Autodesk Fusion 360 part; units mm, degrees
note: some values were not read from the file. Chosen so that the rebuilt part matches the saved one: which bodies a step acts on; which pieces of a blend or face edit are solid. Set by a fixed rule: which sketch regions a step uses.
(part 2 of 4)
  spline S17 degree 5 poles (12.1174, 16.1235) (12.1106, 16.126) (12.0971, 16.1308) (12.0768, 16.138) (12.0498, 16.1475) (12.0159, 16.1592) (11.9821, 16.1707) (11.9483, 16.1819) (11.9145, 16.193) (11.8807, 16.2039) (11.8468, 16.2146) (11.813, 16.225) (11.7792, 16.2353) (11.7454, 16.2454) (11.7116, 16.2552) (11.6778, 16.2649) (11.644, 16.2743) (11.6102, 16.2836) (11.5765, 16.2926) (11.5427, 16.3014) (11.509, 16.31) (11.4752, 16.3184) (11.4415, 16.3266) (11.4078, 16.3346) (11.3741, 16.3423) (11.3405, 16.3499) (11.3068, 16.3572) (11.2732, 16.3643) (11.2396, 16.3712) (11.206, 16.3778) (11.1724, 16.3842) (11.1389, 16.3904) (11.1054, 16.3964) (11.0719, 16.4021) (11.0384, 16.4076) (11.005, 16.4129) (10.9716, 16.418) (10.9382, 16.4228) (10.9049, 16.4273) (10.8716, 16.4316) (10.8383, 16.4357) (10.8051, 16.4395) (10.7719, 16.4431) (10.7388, 16.4464) (10.7057, 16.4495) (10.6726, 16.4523) (10.6396, 16.4548) (10.6066, 16.4571) (10.5737, 16.4591) (10.5409, 16.4608) (10.508, 16.4623) (10.4753, 16.4635) (10.4426, 16.4643) (10.41, 16.4649) (10.3774, 16.4651) (10.345, 16.465) (10.3125, 16.4647) (10.2802, 16.4641) (10.2479, 16.4632) (10.2156, 16.462) (10.1835, 16.4604) (10.1515, 16.4583) (10.1196, 16.4557) (10.0879, 16.4527) (10.0562, 16.4492) (10.0246, 16.4454) (9.9932, 16.4414) (9.9617, 16.4371) (9.9304, 16.4325) (9.8993, 16.4274) (9.8685, 16.4212) (9.8441, 16.4151) (9.8261, 16.4098) (9.8141, 16.4059) (9.8082, 16.4039) knots -1 -1 -1 -1 -1 -1 -0.98571429 -0.97142857 -0.95714286 -0.94285714 -0.92857143 -0.91428571 -0.9 -0.88571429 -0.87142857 -0.85714286 -0.84285714 -0.82857143 -0.81428571 -0.8 -0.78571429 -0.77142857 -0.75714286 -0.74285714 -0.72857143 -0.71428571 -0.7 -0.68571429 -0.67142857 -0.65714286 -0.64285714 -0.62857143 -0.61428571 -0.6 -0.58571429 -0.57142857 -0.55714286 -0.54285714 -0.52857143 -0.51428571 -0.5 -0.48571429 -0.47142857 -0.45714286 -0.44285714 -0.42857143 -0.41428571 -0.4 -0.38571429 -0.37142857 -0.35714286 -0.34285714 -0.32857143 -0.31428571 -0.3 -0.28571429 -0.27142857 -0.25714286 -0.24285714 -0.22857143 -0.21428571 -0.2 -0.18571429 -0.17142857 -0.15714286 -0.14285714 -0.12857143 -0.11428571 -0.1 -0.08571429 -0.07142857 -0.05714286 -0.04285714 -0.02857143 -0.01428571 0 0 0 0 0 0
  line L17 (9.8082, 16.4039) -> (9.5546, 16.3173)
  arc A36 (8.5618, 16.7569) -> (9.5546, 16.3173) centre (9.2961, 17.0744) ccw
  arc A37 (8.5618, 16.7569) -> (8.4802, 16.94) centre (0, 13.0546) ccw
  arc A38 (8.8179, 17.9719) -> (8.4802, 16.94) centre (9.2075, 17.2732) ccw
  line L18 (8.8179, 17.9719) -> (9.0519, 18.1024)
  spline S18 degree 5 poles (9.0519, 18.1024) (9.0574, 18.1055) (9.0683, 18.1117) (9.0843, 18.1216) (9.1051, 18.1357) (9.1304, 18.1544) (9.1551, 18.1741) (9.1794, 18.1943) (9.2036, 18.2148) (9.2276, 18.2355) (9.2516, 18.2564) (9.2753, 18.2776) (9.2989, 18.2992) (9.3221, 18.3211) (9.3451, 18.3435) (9.3678, 18.3663) (9.3902, 18.3895) (9.4125, 18.4129) (9.4346, 18.4365) (9.4566, 18.4604) (9.4783, 18.4845) (9.5, 18.5088) (9.5214, 18.5334) (9.5426, 18.5583) (9.5637, 18.5834) (9.5845, 18.6088) (9.6052, 18.6344) (9.6258, 18.6602) (9.6461, 18.6862) (9.6663, 18.7124) (9.6864, 18.7389) (9.7062, 18.7655) (9.726, 18.7924) (9.7455, 18.8194) (9.7649, 18.8467) (9.7841, 18.8741) (9.8032, 18.9017) (9.8221, 18.9296) (9.8409, 18.9576) (9.8595, 18.9858) (9.8779, 19.0141) (9.8962, 19.0427) (9.9144, 19.0714) (9.9324, 19.1003) (9.9502, 19.1294) (9.9679, 19.1586) (9.9854, 19.188) (10.0028, 19.2176) (10.02, 19.2474) (10.0371, 19.2773) (10.054, 19.3073) (10.0708, 19.3375) (10.0875, 19.3679) (10.1039, 19.3985) (10.1203, 19.4291) (10.1364, 19.46) (10.1525, 19.491) (10.1684, 19.5221) (10.1841, 19.5534) (10.1997, 19.5848) (10.2151, 19.6164) (10.2304, 19.6481) (10.2455, 19.68) (10.2605, 19.712) (10.2754, 19.7441) (10.2901, 19.7764) (10.3046, 19.8088) (10.319, 19.8413) (10.3333, 19.874) (10.3474, 19.9068) (10.3614, 19.9398) (10.3724, 19.9662) (10.3806, 19.9861) (10.3861, 19.9994) (10.3888, 20.0061) knots 0 0 0 0 0 0 0.01428571 0.02857143 0.04285714 0.05714286 0.07142857 0.08571429 0.1 0.11428571 0.12857143 0.14285714 0.15714286 0.17142857 0.18571429 0.2 0.21428571 0.22857143 0.24285714 0.25714286 0.27142857 0.28571429 0.3 0.31428571 0.32857143 0.34285714 0.35714286 0.37142857 0.38571429 0.4 0.41428571 0.42857143 0.44285714 0.45714286 0.47142857 0.48571429 0.5 0.51428571 0.52857143 0.54285714 0.55714286 0.57142857 0.58571429 0.6 0.61428571 0.62857143 0.64285714 0.65714286 0.67142857 0.68571429 0.7 0.71428571 0.72857143 0.74285714 0.75714286 0.77142857 0.78571429 0.8 0.81428571 0.82857143 0.84285714 0.85714286 0.87142857 0.88571429 0.9 0.91428571 0.92857143 0.94285714 0.95714286 0.97142857 0.98571429 1 1 1 1 1 1
  arc A39 (10.3888, 20.0061) -> (9.8216, 20.7868) centre (0, 13.0546) ccw
  spline S19 degree 5 poles (9.8216, 20.7868) (9.8144, 20.7863) (9.8001, 20.7852) (9.7786, 20.7835) (9.75, 20.7812) (9.7144, 20.7781) (9.6788, 20.7748) (9.6433, 20.7714) (9.6079, 20.7677) (9.5726, 20.7639) (9.5374, 20.7599) (9.5022, 20.7557) (9.4671, 20.7514) (9.4322, 20.7468) (9.3973, 20.7421) (9.3625, 20.7371) (9.3278, 20.732) (9.2931, 20.7267) (9.2586, 20.7212) (9.2242, 20.7156) (9.1899, 20.7097) (9.1556, 20.7037) (9.1215, 20.6974) (9.0875, 20.691) (9.0536, 20.6844) (9.0197, 20.6776) (8.986, 20.6706) (8.9524, 20.6634) (8.9189, 20.656) (8.8855, 20.6484) (8.8522, 20.6406) (8.8191, 20.6326) (8.786, 20.6245) (8.7531, 20.6161) (8.7203, 20.6075) (8.6876, 20.5987) (8.6551, 20.5897) (8.6226, 20.5805) (8.5903, 20.5712) (8.5581, 20.5616) (8.5261, 20.5517) (8.4942, 20.5417) (8.4624, 20.5315) (8.4308, 20.521) (8.3993, 20.5104) (8.368, 20.4995) (8.3368, 20.4884) (8.3057, 20.477) (8.2748, 20.4655) (8.2441, 20.4537) (8.2135, 20.4417) (8.1831, 20.4294) (8.1529, 20.4169) (8.1229, 20.4041) (8.0931, 20.3911) (8.0634, 20.3779) (8.034, 20.3644) (8.0046, 20.3506) (7.9755, 20.3367) (7.9465, 20.3225) (7.9179, 20.3079) (7.8895, 20.293) (7.8614, 20.2777) (7.8336, 20.262) (7.8061, 20.2459) (7.7788, 20.2296) (7.7517, 20.2132) (7.7247, 20.1965) (7.698, 20.1796) (7.6717, 20.1622) (7.646, 20.144) (7.6262, 20.1285) (7.6119, 20.1164) (7.6025, 20.1079) (7.5979, 20.1037) knots -1 -1 -1 -1 -1 -1 -0.98571429 -0.97142857 -0.95714286 -0.94285714 -0.92857143 -0.91428571 -0.9 -0.88571429 -0.87142857 -0.85714286 -0.84285714 -0.82857143 -0.81428571 -0.8 -0.78571429 -0.77142857 -0.75714286 -0.74285714 -0.72857143 -0.71428571 -0.7 -0.68571429 -0.67142857 -0.65714286 -0.64285714 -0.62857143 -0.61428571 -0.6 -0.58571429 -0.57142857 -0.55714286 -0.54285714 -0.52857143 -0.51428571 -0.5 -0.48571429 -0.47142857 -0.45714286 -0.44285714 -0.42857143 -0.41428571 -0.4 -0.38571429 -0.37142857 -0.35714286 -0.34285714 -0.32857143 -0.31428571 -0.3 -0.28571429 -0.27142857 -0.25714286 -0.24285714 -0.22857143 -0.21428571 -0.2 -0.18571429 -0.17142857 -0.15714286 -0.14285714 -0.12857143 -0.11428571 -0.1 -0.08571429 -0.07142857 -0.05714286 -0.04285714 -0.02857143 -0.01428571 0 0 0 0 0 0
  line L19 (7.5979, 20.1037) -> (7.4015, 19.9214)
  arc A40 (6.3157, 19.9192) -> (7.4015, 19.9214) centre (6.8574, 20.5079) ccw
  arc A41 (6.3157, 19.9192) -> (6.1668, 20.0533) centre (0, 13.0546) ccw
  arc A42 (6.0555, 21.1333) -> (6.1668, 20.0533) centre (6.6957, 20.6535) ccw
  line L20 (6.0555, 21.1333) -> (6.2162, 21.3477)
  spline S20 degree 5 poles (6.2162, 21.3477) (6.22, 21.3528) (6.2274, 21.3629) (6.238, 21.3785) (6.2513, 21.3998) (6.2667, 21.4272) (6.2813, 21.4552) (6.2953, 21.4835) (6.3091, 21.5121) (6.3226, 21.5408) (6.336, 21.5697) (6.3491, 21.5987) (6.3618, 21.6279) (6.3741, 21.6575) (6.3859, 21.6873) (6.3974, 21.7173) (6.4085, 21.7476) (6.4194, 21.778) (6.4299, 21.8086) (6.4403, 21.8394) (6.4504, 21.8702) (6.4602, 21.9013) (6.4698, 21.9325) (6.4791, 21.9638) (6.4881, 21.9953) (6.4968, 22.027) (6.5053, 22.0588) (6.5136, 22.0907) (6.5216, 22.1228) (6.5294, 22.1549) (6.5369, 22.1872) (6.5443, 22.2197) (6.5514, 22.2522) (6.5582, 22.2849) (6.5649, 22.3177) (6.5713, 22.3505) (6.5774, 22.3836) (6.5834, 22.4167) (6.5891, 22.4499) (6.5947, 22.4832) (6.6, 22.5166) (6.6051, 22.5502) (6.61, 22.5838) (6.6147, 22.6175) (6.6191, 22.6513) (6.6234, 22.6852) (6.6274, 22.7192) (6.6313, 22.7533) (6.6349, 22.7875) (6.6384, 22.8218) (6.6416, 22.8561) (6.6447, 22.8905) (6.6475, 22.925) (6.6501, 22.9596) (6.6526, 22.9943) (6.6548, 23.0291) (6.6568, 23.0639) (6.6587, 23.0988) (6.6603, 23.1338) (6.6618, 23.1688) (6.6631, 23.204) (6.6641, 23.2392) (6.665, 23.2744) (6.6657, 23.3097) (6.6662, 23.3451) (6.6665, 23.3806) (6.6666, 23.4161) (6.6665, 23.4517) (6.6662, 23.4874) (6.6658, 23.5231) (6.6651, 23.5589) (6.6645, 23.5875) (6.6639, 23.609) (6.6634, 23.6234) (6.6632, 23.6306) knots 0 0 0 0 0 0 0.01428571 0.02857143 0.04285714 0.05714286 0.07142857 0.08571429 0.1 0.11428571 0.12857143 0.14285714 0.15714286 0.17142857 0.18571429 0.2 0.21428571 0.22857143 0.24285714 0.25714286 0.27142857 0.28571429 0.3 0.31428571 0.32857143 0.34285714 0.35714286 0.37142857 0.38571429 0.4 0.41428571 0.42857143 0.44285714 0.45714286 0.47142857 0.48571429 0.5 0.51428571 0.52857143 0.54285714 0.55714286 0.57142857 0.58571429 0.6 0.61428571 0.62857143 0.64285714 0.65714286 0.67142857 0.68571429 0.7 0.71428571 0.72857143 0.74285714 0.75714286 0.77142857 0.78571429 0.8 0.81428571 0.82857143 0.84285714 0.85714286 0.87142857 0.88571429 0.9 0.91428571 0.92857143 0.94285714 0.95714286 0.97142857 0.98571429 1 1 1 1 1 1
  arc A43 (6.6632, 23.6306) -> (5.8275, 24.1131) centre (0, 13.0546) ccw
  spline S21 degree 5 poles (5.8275, 24.1131) (5.8211, 24.1097) (5.8085, 24.1029) (5.7895, 24.0927) (5.7644, 24.0789) (5.7331, 24.0616) (5.7019, 24.0441) (5.6709, 24.0265) (5.6401, 24.0088) (5.6093, 23.9909) (5.5788, 23.9729) (5.5484, 23.9548) (5.5181, 23.9366) (5.488, 23.9182) (5.4581, 23.8997) (5.4283, 23.881) (5.3987, 23.8622) (5.3692, 23.8433) (5.3399, 23.8242) (5.3107, 23.8051) (5.2818, 23.7858) (5.2529, 23.7663) (5.2243, 23.7467) (5.1958, 23.727) (5.1675, 23.7072) (5.1394, 23.6872) (5.1115, 23.6671) (5.0837, 23.6468) (5.0561, 23.6265) (5.0287, 23.6059) (5.0014, 23.5853) (4.9744, 23.5645) (4.9475, 23.5436) (4.9208, 23.5226) (4.8944, 23.5014) (4.8681, 23.4801) (4.842, 23.4586) (4.8161, 23.437) (4.7904, 23.4153) (4.7649, 23.3935) (4.7396, 23.3715) (4.7145, 23.3493) (4.6897, 23.327) (4.665, 23.3046) (4.6406, 23.2821) (4.6164, 23.2594) (4.5924, 23.2365) (4.5687, 23.2136) (4.5452, 23.1905) (4.5219, 23.1672) (4.4988, 23.1438) (4.4761, 23.1202) (4.4536, 23.0965) (4.4313, 23.0726) (4.4094, 23.0486) (4.3877, 23.0244) (4.3662, 23.0001) (4.345, 22.9756) (4.3241, 22.951) (4.3034, 22.9263) (4.2831, 22.9013) (4.2633, 22.8761) (4.2438, 22.8507) (4.2249, 22.8251) (4.2063, 22.7992) (4.188, 22.7733) (4.1699, 22.7472) (4.152, 22.721) (4.1345, 22.6946) (4.1175, 22.668) (4.1015, 22.641) (4.0897, 22.6188) (4.0815, 22.6019) (4.0764, 22.5904) (4.0739, 22.5846) knots -1 -1 -1 -1 -1 -1 -0.98571429 -0.97142857 -0.95714286 -0.94285714 -0.92857143 -0.91428571 -0.9 -0.88571429 -0.87142857 -0.85714286 -0.84285714 -0.82857143 -0.81428571 -0.8 -0.78571429 -0.77142857 -0.75714286 -0.74285714 -0.72857143 -0.71428571 -0.7 -0.68571429 -0.67142857 -0.65714286 -0.64285714 -0.62857143 -0.61428571 -0.6 -0.58571429 -0.57142857 -0.55714286 -0.54285714 -0.52857143 -0.51428571 -0.5 -0.48571429 -0.47142857 -0.45714286 -0.44285714 -0.42857143 -0.41428571 -0.4 -0.38571429 -0.37142857 -0.35714286 -0.34285714 -0.32857143 -0.31428571 -0.3 -0.28571429 -0.27142857 -0.25714286 -0.24285714 -0.22857143 -0.21428571 -0.2 -0.18571429 -0.17142857 -0.15714286 -0.14285714 -0.12857143 -0.11428571 -0.1 -0.08571429 -0.07142857 -0.05714286 -0.04285714 -0.02857143 -0.01428571 0 0 0 0 0 0
  line L21 (4.0739, 22.5846) -> (3.9686, 22.3382)
  arc A44 (2.9776, 21.8945) -> (3.9686, 22.3382) centre (3.233, 22.6527) ccw
  arc A45 (2.9776, 21.8945) -> (2.787, 21.9565) centre (0, 13.0546) ccw
  arc A46 (2.2461, 22.8979) -> (2.787, 21.9565) centre (3.026, 22.7199) ccw
  line L22 (2.2461, 22.8979) -> (2.3057, 23.1591)
  spline S22 degree 5 poles (2.3057, 23.1591) (2.3071, 23.1653) (2.3097, 23.1776) (2.3131, 23.1961) (2.3166, 23.2209) (2.3195, 23.2522) (2.3214, 23.2837) (2.3227, 23.3154) (2.3236, 23.347) (2.3244, 23.3788) (2.3248, 23.4106) (2.325, 23.4424) (2.3247, 23.4743) (2.3239, 23.5063) (2.3226, 23.5383) (2.3209, 23.5705) (2.3187, 23.6026) (2.3162, 23.6348) (2.3135, 23.6671) (2.3104, 23.6994) (2.3071, 23.7317) (2.3034, 23.764) (2.2995, 23.7964) (2.2952, 23.8288) (2.2906, 23.8613) (2.2858, 23.8938) (2.2806, 23.9263) (2.2751, 23.9588) (2.2694, 23.9913) (2.2634, 24.0239) (2.2572, 24.0565) (2.2507, 24.0891) (2.244, 24.1217) (2.2369, 24.1543) (2.2297, 24.187) (2.2221, 24.2196) (2.2144, 24.2523) (2.2063, 24.285) (2.1981, 24.3177) (2.1896, 24.3504) (2.1808, 24.3831) (2.1719, 24.4158) (2.1627, 24.4485) (2.1532, 24.4812) (2.1435, 24.5139) (2.1336, 24.5466) (2.1235, 24.5793) (2.1132, 24.612) (2.1026, 24.6447) (2.0918, 24.6774) (2.0808, 24.7101) (2.0696, 24.7428) (2.0581, 24.7755) (2.0465, 24.8082) (2.0346, 24.8408) (2.0225, 24.8735) (2.0102, 24.9061) (1.9977, 24.9388) (1.985, 24.9714) (1.972, 25.004) (1.9589, 25.0366) (1.9455, 25.0692) (1.932, 25.1018) (1.9183, 25.1343) (1.9043, 25.1669) (1.8902, 25.1994) (1.8758, 25.2319) (1.8613, 25.2644) (1.8465, 25.2968) (1.8316, 25.3292) (1.8164, 25.3617) (1.8042, 25.3876) (1.7949, 25.407) (1.7886, 25.42) (1.7855, 25.4264) knots 0 0 0 0 0 0 0.01428571 0.02857143 0.04285714 0.05714286 0.07142857 0.08571429 0.1 0.11428571 0.12857143 0.14285714 0.15714286 0.17142857 0.18571429 0.2 0.21428571 0.22857143 0.24285714 0.25714286 0.27142857 0.28571429 0.3 0.31428571 0.32857143 0.34285714 0.35714286 0.37142857 0.38571429 0.4 0.41428571 0.42857143 0.44285714 0.45714286 0.47142857 0.48571429 0.5 0.51428571 0.52857143 0.54285714 0.55714286 0.57142857 0.58571429 0.6 0.61428571 0.62857143 0.64285714 0.65714286 0.67142857 0.68571429 0.7 0.71428571 0.72857143 0.74285714 0.75714286 0.77142857 0.78571429 0.8 0.81428571 0.82857143 0.84285714 0.85714286 0.87142857 0.88571429 0.9 0.91428571 0.92857143 0.94285714 0.95714286 0.97142857 0.98571429 1 1 1 1 1 1
  arc A47 (1.7855, 25.4264) -> (0.8258, 25.5273) centre (0, 13.0546) ccw
  spline S23 degree 5 poles (0.8258, 25.5273) (0.8214, 25.5216) (0.8126, 25.5103) (0.7994, 25.4932) (0.782, 25.4704) (0.7605, 25.4418) (0.7391, 25.4132) (0.718, 25.3845) (0.697, 25.3558) (0.6762, 25.327) (0.6556, 25.2981) (0.6352, 25.2692) (0.615, 25.2402) (0.5949, 25.2111) (0.5751, 25.182) (0.5555, 25.1529) (0.5361, 25.1237) (0.5168, 25.0944) (0.4978, 25.0651) (0.479, 25.0357) (0.4604, 25.0063) (0.442, 24.9768) (0.4238, 24.9473) (0.4058, 24.9177) (0.388, 24.888) (0.3704, 24.8583) (0.3531, 24.8286) (0.3359, 24.7988) (0.319, 24.769) (0.3023, 24.7391) (0.2858, 24.7091) (0.2695, 24.6792) (0.2535, 24.6491) (0.2377, 24.619) (0.2221, 24.5889) (0.2068, 24.5588) (0.1917, 24.5286) (0.1768, 24.4983) (0.1622, 24.468) (0.1478, 24.4377) (0.1336, 24.4073) (0.1197, 24.3769) (0.1061, 24.3464) (0.0927, 24.3159) (0.0795, 24.2854) (0.0667, 24.2548) (0.054, 24.2242) (0.0417, 24.1935) (0.0296, 24.1629) (0.0178, 24.1321) (0.0062, 24.1014) (-0.005, 24.0706) (-0.0159, 24.0398) (-0.0265, 24.0089) (-0.0368, 23.978) (-0.0467, 23.9471) (-0.0564, 23.9162) (-0.0659, 23.8852) (-0.075, 23.8542) (-0.0838, 23.8232) (-0.0922, 23.7921) (-0.1001, 23.7611) (-0.1075, 23.7299) (-0.1144, 23.6988) (-0.1209, 23.6676) (-0.127, 23.6364) (-0.133, 23.6052) (-0.1386, 23.574) (-0.1439, 23.5429) (-0.1486, 23.5117) (-0.1523, 23.4804) (-0.154, 23.4554) (-0.1546, 23.4366) (-0.1546, 23.424) (-0.1545, 23.4177) knots -1 -1 -1 -1 -1 -1 -0.98571429 -0.97142857 -0.95714286 -0.94285714 -0.92857143 -0.91428571 -0.9 -0.88571429 -0.87142857 -0.85714286 -0.84285714 -0.82857143 -0.81428571 -0.8 -0.78571429 -0.77142857 -0.75714286 -0.74285714 -0.72857143 -0.71428571 -0.7 -0.68571429 -0.67142857 -0.65714286 -0.64285714 -0.62857143 -0.61428571 -0.6 -0.58571429 -0.57142857 -0.55714286 -0.54285714 -0.52857143 -0.51428571 -0.5 -0.48571429 -0.47142857 -0.45714286 -0.44285714 -0.42857143 -0.41428571 -0.4 -0.38571429 -0.37142857 -0.35714286 -0.34285714 -0.32857143 -0.31428571 -0.3 -0.28571429 -0.27142857 -0.25714286 -0.24285714 -0.22857143 -0.21428571 -0.2 -0.18571429 -0.17142857 -0.15714286 -0.14285714 -0.12857143 -0.11428571 -0.1 -0.08571429 -0.07142857 -0.05714286 -0.04285714 -0.02857143 -0.01428571 0 0 0 0 0 0
  line L23 (-0.1545, 23.4177) -> (-0.1505, 23.1498)
  arc A48 (-0.8753, 22.3414) -> (-0.1505, 23.1498) centre (-0.9504, 23.1379) ccw
  arc A49 (-0.8753, 22.3414) -> (-1.0746, 22.3204) centre (0, 13.0546) ccw
  arc A50 (-1.9517, 22.9605) -> (-1.0746, 22.3204) centre (-1.1668, 23.1151) ccw
  line L24 (-1.9517, 22.9605) -> (-2.0035, 23.2234)
  spline S24 degree 5 poles (-2.0035, 23.2234) (-2.0047, 23.2295) (-2.0073, 23.2418) (-2.0118, 23.2601) (-2.0187, 23.2842) (-2.0288, 23.314) (-2.0398, 23.3436) (-2.0515, 23.373) (-2.0636, 23.4023) (-2.0758, 23.4316) (-2.0883, 23.4608) (-2.1011, 23.49) (-2.1144, 23.519) (-2.1281, 23.5479) (-2.1423, 23.5767) (-2.157, 23.6053) (-2.172, 23.6338) (-2.1874, 23.6622) (-2.203, 23.6906) (-2.219, 23.7188) (-2.2352, 23.747) (-2.2516, 23.7751) (-2.2684, 23.803) (-2.2855, 23.8309) (-2.3029, 23.8587) (-2.3205, 23.8864) (-2.3385, 23.914) (-2.3567, 23.9415) (-2.3751, 23.9689) (-2.3939, 23.9962) (-2.4128, 24.0234) (-2.432, 24.0506) (-2.4514, 24.0776) (-2.4711, 24.1046) (-2.491, 24.1314) (-2.5112, 24.1582) (-2.5316, 24.1849) (-2.5522, 24.2115) (-2.5731, 24.238) (-2.5941, 24.2644) (-2.6154, 24.2907) (-2.6369, 24.3169) (-2.6586, 24.343) (-2.6805, 24.3691) (-2.7027, 24.395) (-2.725, 24.4209) (-2.7476, 24.4467) (-2.7703, 24.4723) (-2.7933, 24.4979) (-2.8165, 24.5234) (-2.8398, 24.5488) (-2.8634, 24.5741) (-2.8871, 24.5993) (-2.9111, 24.6244) (-2.9352, 24.6494) (-2.9595, 24.6743) (-2.9841, 24.6991) (-3.0088, 24.7239) (-3.0337, 24.7485) (-3.0587, 24.773) (-3.084, 24.7975) (-3.1094, 24.8218) (-3.135, 24.846) (-3.1608, 24.8702) (-3.1868, 24.8942) (-3.213, 24.9182) (-3.2393, 24.9421) (-3.2658, 24.9658) (-3.2925, 24.9895) (-3.3193, 25.013) (-3.3463, 25.0365) (-3.3681, 25.0552) (-3.3845, 25.0691) (-3.3954, 25.0784) (-3.4009, 25.0831) knots 0 0 0 0 0 0 0.01428571 0.02857143 0.04285714 0.05714286 0.07142857 0.08571429 0.1 0.11428571 0.12857143 0.14285714 0.15714286 0.17142857 0.18571429 0.2 0.21428571 0.22857143 0.24285714 0.25714286 0.27142857 0.28571429 0.3 0.31428571 0.32857143 0.34285714 0.35714286 0.37142857 0.38571429 0.4 0.41428571 0.42857143 0.44285714 0.45714286 0.47142857 0.48571429 0.5 0.51428571 0.52857143 0.54285714 0.55714286 0.57142857 0.58571429 0.6 0.61428571 0.62857143 0.64285714 0.65714286 0.67142857 0.68571429 0.7 0.71428571 0.72857143 0.74285714 0.75714286 0.77142857 0.78571429 0.8 0.81428571 0.82857143 0.84285714 0.85714286 0.87142857 0.88571429 0.9 0.91428571 0.92857143 0.94285714 0.95714286 0.97142857 0.98571429 1 1 1 1 1 1
  arc A51 (-3.4009, 25.0831) -> (-4.3187, 24.7848) centre (0, 13.0546) ccw
  spline S25 degree 5 poles (-4.3187, 24.7848) (-4.3205, 24.7779) (-4.3239, 24.7639) (-4.3289, 24.743) (-4.3355, 24.7151) (-4.3436, 24.6802) (-4.3515, 24.6454) (-4.3591, 24.6106) (-4.3666, 24.5758) (-4.3739, 24.541) (-4.381, 24.5062) (-4.3879, 24.4715) (-4.3945, 24.4368) (-4.401, 24.4021) (-4.4073, 24.3675) (-4.4133, 24.3329) (-4.4192, 24.2983) (-4.4249, 24.2637) (-4.4303, 24.2292) (-4.4356, 24.1947) (-4.4406, 24.1603) (-4.4454, 24.1258) (-4.45, 24.0914) (-4.4544, 24.0571) (-4.4586, 24.0228) (-4.4626, 23.9885) (-4.4664, 23.9543) (-4.4699, 23.9201) (-4.4732, 23.886) (-4.4763, 23.8519) (-4.4792, 23.8178) (-4.4819, 23.7838) (-4.4843, 23.7498) (-4.4865, 23.7159) (-4.4885, 23.6821) (-4.4903, 23.6483) (-4.4918, 23.6145) (-4.4931, 23.5808) (-4.4941, 23.5472) (-4.4949, 23.5136) (-4.4955, 23.4801) (-4.4958, 23.4467) (-4.4959, 23.4133) (-4.4957, 23.38) (-4.4953, 23.3468) (-4.4946, 23.3136) (-4.4937, 23.2805) (-4.4925, 23.2475) (-4.4911, 23.2145) (-4.4894, 23.1817) (-4.4874, 23.1489) (-4.4852, 23.1162) (-4.4826, 23.0836) (-4.4797, 23.0511) (-4.4765, 23.0187) (-4.4731, 22.9864) (-4.4694, 22.9542) (-4.4654, 22.9221) (-4.4611, 22.89) (-4.4565, 22.8581) (-4.4516, 22.8263) (-4.4461, 22.7947) (-4.4403, 22.7633) (-4.4339, 22.732) (-4.4271, 22.7009) (-4.4201, 22.6699) (-4.4128, 22.639) (-4.4053, 22.6082) (-4.3974, 22.5776) (-4.389, 22.5471) (-4.3796, 22.5171) (-4.3711, 22.4935) (-4.3639, 22.4761) (-4.3588, 22.4647) (-4.3562, 22.4589) knots -1 -1 -1 -1 -1 -1 -0.98571429 -0.97142857 -0.95714286 -0.94285714 -0.92857143 -0.91428571 -0.9 -0.88571429 -0.87142857 -0.85714286 -0.84285714 -0.82857143 -0.81428571 -0.8 -0.78571429 -0.77142857 -0.75714286 -0.74285714 -0.72857143 -0.71428571 -0.7 -0.68571429 -0.67142857 -0.65714286 -0.64285714 -0.62857143 -0.61428571 -0.6 -0.58571429 -0.57142857 -0.55714286 -0.54285714 -0.52857143 -0.51428571 -0.5 -0.48571429 -0.47142857 -0.45714286 -0.44285714 -0.42857143 -0.41428571 -0.4 -0.38571429 -0.37142857 -0.35714286 -0.34285714 -0.32857143 -0.31428571 -0.3 -0.28571429 -0.27142857 -0.25714286 -0.24285714 -0.22857143 -0.21428571 -0.2 -0.18571429 -0.17142857 -0.15714286 -0.14285714 -0.12857143 -0.11428571 -0.1 -0.08571429 -0.07142857 -0.05714286 -0.04285714 -0.02857143 -0.01428571 0 0 0 0 0 0
  line L25 (-4.3562, 22.4589) -> (-4.2435, 22.2158)
  arc A52 (-4.5769, 21.1825) -> (-4.2435, 22.2158) centre (-4.9694, 21.8796) ccw
  arc A53 (-4.5769, 21.1825) -> (-4.7505, 21.0823) centre (0, 13.0546) ccw
  arc A54 (-5.8121, 21.3102) -> (-4.7505, 21.0823) centre (-5.1579, 21.7708) ccw
  line L26 (-5.8121, 21.3102) -> (-5.9663, 21.5293)
  spline S26 degree 5 poles (-5.9663, 21.5293) (-5.9699, 21.5345) (-5.9773, 21.5446) (-5.9888, 21.5595) (-6.005, 21.5788) (-6.0263, 21.6019) (-6.0484, 21.6244) (-6.071, 21.6465) (-6.0939, 21.6684) (-6.1171, 21.6902) (-6.1404, 21.7118) (-6.1639, 21.7332) (-6.1878, 21.7543) (-6.2121, 21.7751) (-6.2368, 21.7956) (-6.2618, 21.8158) (-6.2872, 21.8358) (-6.3128, 21.8555) (-6.3386, 21.875) (-6.3646, 21.8943) (-6.3909, 21.9134) (-6.4174, 21.9324) (-6.4441, 21.9511) (-6.471, 21.9697) (-6.4982, 21.988) (-6.5256, 22.0061) (-6.5532, 22.024) (-6.581, 22.0417) (-6.609, 22.0592) (-6.6372, 22.0766) (-6.6656, 22.0937) (-6.6942, 22.1107) (-6.723, 22.1275) (-6.7519, 22.1442) (-6.781, 22.1606) (-6.8103, 22.1768) (-6.8398, 22.1929) (-6.8695, 22.2088) (-6.8993, 22.2246) (-6.9293, 22.2401) (-6.9594, 22.2555) (-6.9897, 22.2707) (-7.0202, 22.2858) (-7.0508, 22.3006) (-7.0816, 22.3153) (-7.1125, 22.3299) (-7.1436, 22.3442) (-7.1748, 22.3584) (-7.2062, 22.3724) (-7.2377, 22.3863) (-7.2694, 22.4) (-7.3012, 22.4135) (-7.3332, 22.4269) (-7.3652, 22.4401) (-7.3975, 22.4531) (-7.4298, 22.466) (-7.4623, 22.4787) (-7.495, 22.4912) (-7.5277, 22.5036) (-7.5606, 22.5158) (-7.5936, 22.5279) (-7.6267, 22.5398) (-7.66, 22.5515) (-7.6934, 22.5631) (-7.7269, 22.5745) (-7.7606, 22.5857) (-7.7943, 22.5968) (-7.8282, 22.6077) (-7.8622, 22.6185) (-7.8963, 22.6291) (-7.9305, 22.6395) (-7.958, 22.6477) (-7.9786, 22.6538) (-7.9924, 22.6579) (-7.9993, 22.6599) knots 0 0 0 0 0 0 0.01428571 0.02857143 0.04285714 0.05714286 0.07142857 0.08571429 0.1 0.11428571 0.12857143 0.14285714 0.15714286 0.17142857 0.18571429 0.2 0.21428571 0.22857143 0.24285714 0.25714286 0.27142857 0.28571429 0.3 0.31428571 0.32857143 0.34285714 0.35714286 0.37142857 0.38571429 0.4 0.41428571 0.42857143 0.44285714 0.45714286 0.47142857 0.48571429 0.5 0.51428571 0.52857143 0.54285714 0.55714286 0.57142857 0.58571429 0.6 0.61428571 0.62857143 0.64285714 0.65714286 0.67142857 0.68571429 0.7 0.71428571 0.72857143 0.74285714 0.75714286 0.77142857 0.78571429 0.8 0.81428571 0.82857143 0.84285714 0.85714286 0.87142857 0.88571429 0.9 0.91428571 0.92857143 0.94285714 0.95714286 0.97142857 0.98571429 1 1 1 1 1 1
  arc A55 (-7.9993, 22.6599) -> (-8.7165, 22.0141) centre (0, 13.0546) ccw
  spline S27 degree 5 poles (-8.7165, 22.0141) (-8.7152, 22.0071) (-8.7126, 21.9929) (-8.7087, 21.9717) (-8.7034, 21.9436) (-8.6966, 21.9084) (-8.6896, 21.8734) (-8.6825, 21.8385) (-8.6752, 21.8036) (-8.6677, 21.7689) (-8.66, 21.7343) (-8.6522, 21.6998) (-8.6442, 21.6654) (-8.636, 21.631) (-8.6276, 21.5968) (-8.6191, 21.5628) (-8.6104, 21.5288) (-8.6015, 21.4949) (-8.5924, 21.4611) (-8.5832, 21.4275) (-8.5738, 21.394) (-8.5642, 21.3606) (-8.5544, 21.3273) (-8.5445, 21.2941) (-8.5343, 21.261) (-8.524, 21.2281) (-8.5135, 21.1953) (-8.5029, 21.1626) (-8.492, 21.1301) (-8.481, 21.0977) (-8.4698, 21.0654) (-8.4584, 21.0333) (-8.4468, 21.0013) (-8.435, 20.9694) (-8.423, 20.9376) (-8.4109, 20.9061) (-8.3985, 20.8746) (-8.386, 20.8433) (-8.3733, 20.8122) (-8.3604, 20.7812) (-8.3473, 20.7503) (-8.334, 20.7196) (-8.3205, 20.6891) (-8.3068, 20.6588) (-8.2929, 20.6286) (-8.2788, 20.5985) (-8.2645, 20.5687) (-8.2499, 20.539) (-8.2352, 20.5095) (-8.2203, 20.4801) (-8.2052, 20.451) (-8.1898, 20.422) (-8.1742, 20.3933) (-8.1584, 20.3648) (-8.1423, 20.3365) (-8.126, 20.3084) (-8.1095, 20.2805) (-8.0928, 20.2527) (-8.0759, 20.2252) (-8.0587, 20.1979) (-8.0412, 20.1709) (-8.0234, 20.1442) (-8.0053, 20.1179) (-7.9867, 20.0919) (-7.9679, 20.0663) (-7.9488, 20.0408) (-7.9296, 20.0156) (-7.9102, 19.9905) (-7.8906, 19.9657) (-7.8705, 19.9413) (-7.8498, 19.9177) (-7.8323, 19.8996) (-7.8187, 19.8866) (-7.8094, 19.8782) (-7.8046, 19.8741) knots -1 -1 -1 -1 -1 -1 -0.98571429 -0.97142857 -0.95714286 -0.94285714 -0.92857143 -0.91428571 -0.9 -0.88571429 -0.87142857 -0.85714286 -0.84285714 -0.82857143 -0.81428571 -0.8 -0.78571429 -0.77142857 -0.75714286 -0.74285714 -0.72857143 -0.71428571 -0.7 -0.68571429 -0.67142857 -0.65714286 -0.64285714 -0.62857143 -0.61428571 -0.6 -0.58571429 -0.57142857 -0.55714286 -0.54285714 -0.52857143 -0.51428571 -0.5 -0.48571429 -0.47142857 -0.45714286 -0.44285714 -0.42857143 -0.41428571 -0.4 -0.38571429 -0.37142857 -0.35714286 -0.34285714 -0.32857143 -0.31428571 -0.3 -0.28571429 -0.27142857 -0.25714286 -0.24285714 -0.22857143 -0.21428571 -0.2 -0.18571429 -0.17142857 -0.15714286 -0.14285714 -0.12857143 -0.11428571 -0.1 -0.08571429 -0.07142857 -0.05714286 -0.04285714 -0.02857143 -0.01428571 0 0 0 0 0 0
  line L27 (-7.8046, 19.8741) -> (-7.6029, 19.6978)
  arc A56 (-7.4871, 18.6182) -> (-7.6029, 19.6978) centre (-8.1292, 19.0953) ccw
  arc A57 (-7.4871, 18.6182) -> (-7.6049, 18.456) centre (0, 13.0546) ccw
  arc A58 (-8.6674, 18.2325) -> (-7.6049, 18.456) centre (-8.2572, 18.9193) ccw
  line L28 (-8.6674, 18.2325) -> (-8.8975, 18.3699)
  spline S28 degree 5 poles (-8.8975, 18.3699) (-8.9029, 18.3732) (-8.9137, 18.3794) (-8.9303, 18.3884) (-8.9529, 18.3994) (-8.9818, 18.4118) (-9.0111, 18.4234) (-9.0408, 18.4344) (-9.0706, 18.4451) (-9.1006, 18.4555) (-9.1307, 18.4658) (-9.1609, 18.4758) (-9.1914, 18.4854) (-9.222, 18.4945) (-9.2529, 18.5032) (-9.284, 18.5115) (-9.3152, 18.5194) (-9.3466, 18.527) (-9.3782, 18.5343) (-9.4098, 18.5413) (-9.4416, 18.5482) (-9.4735, 18.5547) (-9.5055, 18.5609) (-9.5376, 18.5669) (-9.5699, 18.5726) (-9.6023, 18.578) (-9.6348, 18.5831) (-9.6674, 18.588) (-9.7002, 18.5926) (-9.733, 18.597) (-9.7659, 18.6011) (-9.7989, 18.605) (-9.832, 18.6087) (-9.8652, 18.6121) (-9.8985, 18.6152) (-9.9319, 18.6182) (-9.9654, 18.6209) (-9.9989, 18.6233) (-10.0326, 18.6256) (-10.0663, 18.6276) (-10.1001, 18.6294) (-10.134, 18.631) (-10.1679, 18.6323) (-10.2019, 18.6334) (-10.236, 18.6344) (-10.2702, 18.635) (-10.3044, 18.6355) (-10.3387, 18.6358) (-10.3731, 18.6358) (-10.4075, 18.6357) (-10.442, 18.6353) (-10.4766, 18.6347) (-10.5112, 18.6339) (-10.5459, 18.6329) (-10.5806, 18.6317) (-10.6154, 18.6303) (-10.6503, 18.6287) (-10.6852, 18.6269) (-10.7202, 18.6249) (-10.7552, 18.6227) (-10.7902, 18.6203) (-10.8253, 18.6176) (-10.8605, 18.6148) (-10.8957, 18.6118) (-10.931, 18.6086) (-10.9663, 18.6052) (-11.0016, 18.6016) (-11.037, 18.5978) (-11.0724, 18.5938) (-11.1079, 18.5896) (-11.1434, 18.5852) (-11.1718, 18.5816) (-11.1932, 18.5787) (-11.2074, 18.5768) (-11.2145, 18.5758) knots 0 0 0 0 0 0 0.01428571 0.02857143 0.04285714 0.05714286 0.07142857 0.08571429 0.1 0.11428571 0.12857143 0.14285714 0.15714286 0.17142857 0.18571429 0.2 0.21428571 0.22857143 0.24285714 0.25714286 0.27142857 0.28571429 0.3 0.31428571 0.32857143 0.34285714 0.35714286 0.37142857 0.38571429 0.4 0.41428571 0.42857143 0.44285714 0.45714286 0.47142857 0.48571429 0.5 0.51428571 0.52857143 0.54285714 0.55714286 0.57142857 0.58571429 0.6 0.61428571 0.62857143 0.64285714 0.65714286 0.67142857 0.68571429 0.7 0.71428571 0.72857143 0.74285714 0.75714286 0.77142857 0.78571429 0.8 0.81428571 0.82857143 0.84285714 0.85714286 0.87142857 0.88571429 0.9 0.91428571 0.92857143 0.94285714 0.95714286 0.97142857 0.98571429 1 1 1 1 1 1
  arc A59 (-11.2145, 18.5758) -> (-11.6071, 17.6942) centre (0, 13.0546) ccw
  spline S29 degree 5 poles (-11.6071, 17.6942) (-11.603, 17.6883) (-11.5949, 17.6764) (-11.5827, 17.6586) (-11.5664, 17.6351) (-11.5459, 17.6057) (-11.5253, 17.5766) (-11.5046, 17.5476) (-11.4837, 17.5187) (-11.4628, 17.4901) (-11.4417, 17.4616) (-11.4205, 17.4332) (-11.3991, 17.405) (-11.3777, 17.377) (-11.3562, 17.3492) (-11.3345, 17.3215) (-11.3127, 17.294) (-11.2908, 17.2667) (-11.2688, 17.2395) (-11.2467, 17.2125) (-11.2244, 17.1857) (-11.2021, 17.1591) (-11.1796, 17.1327) (-11.157, 17.1064) (-11.1344, 17.0803) (-11.1115, 17.0545) (-11.0886, 17.0288) (-11.0656, 17.0032) (-11.0424, 16.9779) (-11.0192, 16.9528) (-10.9958, 16.9279) (-10.9723, 16.9031) (-10.9487, 16.8786) (-10.925, 16.8543) (-10.9011, 16.8302) (-10.8772, 16.8063) (-10.8531, 16.7825) (-10.829, 16.759) (-10.8047, 16.7358) (-10.7803, 16.7127) (-10.7558, 16.6898) (-10.7311, 16.6672) (-10.7064, 16.6448) (-10.6815, 16.6227) (-10.6565, 16.6007) (-10.6314, 16.5791) (-10.6062, 16.5576) (-10.5809, 16.5364) (-10.5554, 16.5154) (-10.5299, 16.4947) (-10.5042, 16.4742) (-10.4784, 16.454) (-10.4524, 16.4341) (-10.4264, 16.4145) (-10.4002, 16.3952) (-10.3738, 16.3761) (-10.3474, 16.3573) (-10.3209, 16.3388) (-10.2942, 16.3205) (-10.2674, 16.3026) (-10.2405, 16.285) (-10.2134, 16.2679) (-10.1861, 16.2512) (-10.1586, 16.235) (-10.1309, 16.2192) (-10.1032, 16.2037) (-10.0753, 16.1885) (-10.0474, 16.1735) (-10.0194, 16.1588) (-9.9912, 16.1447) (-9.9626, 16.1316) (-9.9393, 16.1221) (-9.9216, 16.1158) (-9.9096, 16.1119) (-9.9036, 16.1101) knots -1 -1 -1 -1 -1 -1 -0.98571429 -0.97142857 -0.95714286 -0.94285714 -0.92857143 -0.91428571 -0.9 -0.88571429 -0.87142857 -0.85714286 -0.84285714 -0.82857143 -0.81428571 -0.8 -0.78571429 -0.77142857 -0.75714286 -0.74285714 -0.72857143 -0.71428571 -0.7 -0.68571429 -0.67142857 -0.65714286 -0.64285714 -0.62857143 -0.61428571 -0.6 -0.58571429 -0.57142857 -0.55714286 -0.54285714 -0.52857143 -0.51428571 -0.5 -0.48571429 -0.47142857 -0.45714286 -0.44285714 -0.42857143 -0.41428571 -0.4 -0.38571429 -0.37142857 -0.35714286 -0.34285714 -0.32857143 -0.31428571 -0.3 -0.28571429 -0.27142857 -0.25714286 -0.24285714 -0.22857143 -0.21428571 -0.2 -0.18571429 -0.17142857 -0.15714286 -0.14285714 -0.12857143 -0.11428571 -0.1 -0.08571429 -0.07142857 -0.05714286 -0.04285714 -0.02857143 -0.01428571 0 0 0 0 0 0
  line L29 (-9.9036, 16.1101) -> (-9.6476, 16.0311)
  arc A60 (-9.1027, 15.0919) -> (-9.6476, 16.0311) centre (-9.8834, 15.2666) ccw
extrude "Extrude8" cut sketch "Sketch7" along normal blind 25 contours A0 bodies 1 makes body 2 at (-1.8603, -53.3333, 13.789)
delete_face "DeleteFace1" 1 faces at (-1.8603, -53.3333, 13.789) on bodies 2
move_body "Move6" bodies 1 to x (1, 0, 0) y (0, 1, 0) z (0, 0, 1) at (0, -25, 0)
copy_body "CopyPasteBodies1" bodies 1 makes body 3
move_body "Move7" bodies 3 to x (-1, 0, 0) y (0, -1, 0) z (0, 0, 1) at (-4, 10, 0)
move_body "Move8" bodies 3 to x (1, 0, 0) y (0, 1, 0) z (0, 0, 1) at (4, -10, 0)
extrude "Extrude9" cut 1 faces at (-0.1483, 5, 12.35) along direction (0, 1, 0) blind 30 on bodies 1 bodies 1
move_body "Move9" bodies 2 to x (1, 0, 0) y (0, 1, 0) z (0, 0, 1) at (0, 30, 0)
extrude "Extrude10" add 1 faces at (0.1483, -5, 12.35) along direction (0, 1, 0) blind 30 on bodies 3 bodies 2 3
move_body "Move10" bodies 1 to x (1, 0, 0) y (0, 1, 0) z (0, 0, 1) at (0, 4, 0)
extrude "Extrude11" cut 1 faces at (-0.551, 49, 11.9624) along direction (0, -1, 0) blind 10 on bodies 1 bodies 1
move_body "Move11" bodies 1 to x (1, 0, 0) y (0, 1, 0) z (0, 0, 1) at (0, 1, 0)
extrude "Extrude12" add 1 faces at (-0.2877, 40, 12.9616) along direction (0, -1, 0) blind 4 on bodies 1 bodies 1
sketch "Sketch8" plane through (0, 35, 0) normal (0, 1, 0) x (-1, 0, 0)
  arc A0 (-9.1027, 15.0919) -> (-9.1444, 14.8959) centre (0, 13.0546) ccw
  arc A1 (-10.0241, 14.2595) -> (-9.1444, 14.8959) centre (-9.9287, 15.0538) ccw
  line L0 (-10.0241, 14.2595) -> (-10.2902, 14.2915)
  spline S0 degree 5 poles (-10.2902, 14.2915) (-10.2964, 14.2922) (-10.3089, 14.2935) (-10.3277, 14.295) (-10.3528, 14.2958) (-10.3842, 14.2955) (-10.4157, 14.2941) (-10.4473, 14.2921) (-10.4789, 14.2897) (-10.5106, 14.2871) (-10.5422, 14.2842) (-10.5739, 14.281) (-10.6056, 14.2774) (-10.6373, 14.2733) (-10.6691, 14.2687) (-10.7008, 14.2636) (-10.7326, 14.2581) (-10.7644, 14.2522) (-10.7962, 14.2461) (-10.828, 14.2397) (-10.8597, 14.233) (-10.8915, 14.226) (-10.9233, 14.2187) (-10.9551, 14.211) (-10.9869, 14.2031) (-11.0187, 14.1948) (-11.0505, 14.1863) (-11.0823, 14.1775) (-11.114, 14.1684) (-11.1458, 14.1591) (-11.1776, 14.1494) (-11.2093, 14.1396) (-11.241, 14.1295) (-11.2727, 14.1191) (-11.3045, 14.1084) (-11.3361, 14.0975) (-11.3678, 14.0864) (-11.3995, 14.075) (-11.4311, 14.0633) (-11.4627, 14.0515) (-11.4943, 14.0394) (-11.5259, 14.027) (-11.5575, 14.0144) (-11.589, 14.0016) (-11.6206, 13.9886) (-11.6521, 13.9753) (-11.6835, 13.9618) (-11.715, 13.9481) (-11.7464, 13.9342) (-11.7778, 13.92) (-11.8091, 13.9057) (-11.8405, 13.8911) (-11.8718, 13.8763) (-11.9031, 13.8613) (-11.9343, 13.846) (-11.9655, 13.8306) (-11.9967, 13.815) (-12.0279, 13.7991) (-12.059, 13.783) (-12.0901, 13.7668) (-12.1211, 13.7503) (-12.1521, 13.7336) (-12.1831, 13.7168) (-12.214, 13.6997) (-12.2449, 13.6824) (-12.2758, 13.6649) (-12.3066, 13.6473) (-12.3374, 13.6294) (-12.3682, 13.6113) (-12.3988, 13.5931) (-12.4295, 13.5746) (-12.454, 13.5597) (-12.4723, 13.5485) (-12.4846, 13.5409) (-12.4907, 13.5371) knots 0 0 0 0 0 0 0.01428571 0.02857143 0.04285714 0.05714286 0.07142857 0.08571429 0.1 0.11428571 0.12857143 0.14285714 0.15714286 0.17142857 0.18571429 0.2 0.21428571 0.22857143 0.24285714 0.25714286 0.27142857 0.28571429 0.3 0.31428571 0.32857143 0.34285714 0.35714286 0.37142857 0.38571429 0.4 0.41428571 0.42857143 0.44285714 0.45714286 0.47142857 0.48571429 0.5 0.51428571 0.52857143 0.54285714 0.55714286 0.57142857 0.58571429 0.6 0.61428571 0.62857143 0.64285714 0.65714286 0.67142857 0.68571429 0.7 0.71428571 0.72857143 0.74285714 0.75714286 0.77142857 0.78571429 0.8 0.81428571 0.82857143 0.84285714 0.85714286 0.87142857 0.88571429 0.9 0.91428571 0.92857143 0.94285714 0.95714286 0.97142857 0.98571429 1 1 1 1 1 1
  arc A2 (-12.4907, 13.5371) -> (-12.4907, 12.5721) centre (0, 13.0546) ccw
  spline S1 degree 5 poles (-12.4907, 12.5721) (-12.4846, 12.5683) (-12.4723, 12.5608) (-12.454, 12.5495) (-12.4295, 12.5346) (-12.3988, 12.5161) (-12.3682, 12.4979) (-12.3374, 12.4798) (-12.3066, 12.4619) (-12.2758, 12.4443) (-12.2449, 12.4268) (-12.214, 12.4095) (-12.1831, 12.3925) (-12.1521, 12.3756) (-12.1211, 12.3589) (-12.0901, 12.3424) (-12.059, 12.3262) (-12.0279, 12.3101) (-11.9967, 12.2943) (-11.9655, 12.2786) (-11.9343, 12.2632) (-11.9031, 12.2479) (-11.8718, 12.2329) (-11.8405, 12.2181) (-11.8091, 12.2035) (-11.7778, 12.1892) (-11.7464, 12.175) (-11.715, 12.1611) (-11.6835, 12.1474) (-11.6521, 12.1339) (-11.6206, 12.1206) (-11.589, 12.1076) (-11.5575, 12.0948) (-11.5259, 12.0822) (-11.4943, 12.0699) (-11.4627, 12.0578) (-11.4311, 12.0459) (-11.3995, 12.0342) (-11.3678, 12.0229) (-11.3361, 12.0117) (-11.3045, 12.0008) (-11.2727, 11.9902) (-11.241, 11.9798) (-11.2093, 11.9696) (-11.1776, 11.9598) (-11.1458, 11.9502) (-11.114, 11.9408) (-11.0823, 11.9317) (-11.0505, 11.9229) (-11.0187, 11.9144) (-10.9869, 11.9061) (-10.9551, 11.8982) (-10.9233, 11.8905) (-10.8915, 11.8832) (-10.8597, 11.8762) (-10.828, 11.8696) (-10.7962, 11.8631) (-10.7644, 11.857) (-10.7326, 11.8512) (-10.7008, 11.8457) (-10.6691, 11.8406) (-10.6373, 11.8359) (-10.6056, 11.8318) (-10.5739, 11.8282) (-10.5422, 11.825) (-10.5106, 11.8222) (-10.4789, 11.8195) (-10.4473, 11.8172) (-10.4157, 11.8151) (-10.3842, 11.8138) (-10.3528, 11.8134) (-10.3277, 11.8143) (-10.3089, 11.8157) (-10.2964, 11.817) (-10.2902, 11.8177) knots -1 -1 -1 -1 -1 -1 -0.98571429 -0.97142857 -0.95714286 -0.94285714 -0.92857143 -0.91428571 -0.9 -0.88571429 -0.87142857 -0.85714286 -0.84285714 -0.82857143 -0.81428571 -0.8 -0.78571429 -0.77142857 -0.75714286 -0.74285714 -0.72857143 -0.71428571 -0.7 -0.68571429 -0.67142857 -0.65714286 -0.64285714 -0.62857143 -0.61428571 -0.6 -0.58571429 -0.57142857 -0.55714286 -0.54285714 -0.52857143 -0.51428571 -0.5 -0.48571429 -0.47142857 -0.45714286 -0.44285714 -0.42857143 -0.41428571 -0.4 -0.38571429 -0.37142857 -0.35714286 -0.34285714 -0.32857143 -0.31428571 -0.3 -0.28571429 -0.27142857 -0.25714286 -0.24285714 -0.22857143 -0.21428571 -0.2 -0.18571429 -0.17142857 -0.15714286 -0.14285714 -0.12857143 -0.11428571 -0.1 -0.08571429 -0.07142857 -0.05714286 -0.04285714 -0.02857143 -0.01428571 0 0 0 0 0 0
  line L1 (-10.2902, 11.8177) -> (-10.0241, 11.8497)
  arc A3 (-9.1444, 11.2134) -> (-10.0241, 11.8497) centre (-9.9287, 11.0554) ccw
  arc A4 (-9.1444, 11.2134) -> (-9.1027, 11.0173) centre (0, 13.0546) ccw
  arc A5 (-9.6476, 10.0781) -> (-9.1027, 11.0173) centre (-9.8834, 10.8426) ccw
  line L2 (-9.6476, 10.0781) -> (-9.9036, 9.9991)
  spline S2 degree 5 poles (-9.9036, 9.9991) (-9.9096, 9.9973) (-9.9216, 9.9934) (-9.9393, 9.9871) (-9.9626, 9.9777) (-9.9912, 9.9645) (-10.0194, 9.9505) (-10.0474, 9.9358) (-10.0753, 9.9207) (-10.1032, 9.9055) (-10.1309, 9.89) (-10.1586, 9.8742) (-10.1861, 9.858) (-10.2134, 9.8413) (-10.2405, 9.8242) (-10.2674, 9.8066) (-10.2942, 9.7887) (-10.3209, 9.7704) (-10.3474, 9.7519) (-10.3738, 9.7331) (-10.4002, 9.714) (-10.4264, 9.6947) (-10.4524, 9.6751) (-10.4784, 9.6552) (-10.5042, 9.635) (-10.5299, 9.6146) (-10.5554, 9.5938) (-10.5809, 9.5728) (-10.6062, 9.5516) (-10.6314, 9.5302) (-10.6565, 9.5085) (-10.6815, 9.4865) (-10.7064, 9.4644) (-10.7311, 9.442) (-10.7558, 9.4194) (-10.7803, 9.3965) (-10.8047, 9.3735) (-10.829, 9.3502) (-10.8531, 9.3267) (-10.8772, 9.303) (-10.9011, 9.279) (-10.925, 9.2549) (-10.9487, 9.2306) (-10.9723, 9.2061) (-10.9958, 9.1813) (-11.0192, 9.1564) (-11.0424, 9.1313) (-11.0656, 9.106) (-11.0886, 9.0805) (-11.1115, 9.0548) (-11.1344, 9.0289) (-11.157, 9.0028) (-11.1796, 8.9766) (-11.2021, 8.9501) (-11.2244, 8.9235) (-11.2467, 8.8967) (-11.2688, 8.8697) (-11.2908, 8.8426) (-11.3127, 8.8152) (-11.3345, 8.7877) (-11.3562, 8.7601) (-11.3777, 8.7322) (-11.3991, 8.7042) (-11.4205, 8.676) (-11.4417, 8.6477) (-11.4628, 8.6192) (-11.4837, 8.5905) (-11.5046, 8.5616) (-11.5253, 8.5326) (-11.5459, 8.5035) (-11.5664, 8.4742) (-11.5827, 8.4506) (-11.5949, 8.4328) (-11.603, 8.4209) (-11.6071, 8.415) knots 0 0 0 0 0 0 0.01428571 0.02857143 0.04285714 0.05714286 0.07142857 0.08571429 0.1 0.11428571 0.12857143 0.14285714 0.15714286 0.17142857 0.18571429 0.2 0.21428571 0.22857143 0.24285714 0.25714286 0.27142857 0.28571429 0.3 0.31428571 0.32857143 0.34285714 0.35714286 0.37142857 0.38571429 0.4 0.41428571 0.42857143 0.44285714 0.45714286 0.47142857 0.48571429 0.5 0.51428571 0.52857143 0.54285714 0.55714286 0.57142857 0.58571429 0.6 0.61428571 0.62857143 0.64285714 0.65714286 0.67142857 0.68571429 0.7 0.71428571 0.72857143 0.74285714 0.75714286 0.77142857 0.78571429 0.8 0.81428571 0.82857143 0.84285714 0.85714286 0.87142857 0.88571429 0.9 0.91428571 0.92857143 0.94285714 0.95714286 0.97142857 0.98571429 1 1 1 1 1 1
  arc A6 (-11.6071, 8.415) -> (-11.2145, 7.5334) centre (0, 13.0546) ccw
  spline S3 degree 5 poles (-11.2145, 7.5334) (-11.2074, 7.5324) (-11.1932, 7.5305) (-11.1718, 7.5277) (-11.1434, 7.524) (-11.1079, 7.5196) (-11.0724, 7.5154) (-11.037, 7.5114) (-11.0016, 7.5076) (-10.9663, 7.504) (-10.931, 7.5006) (-10.8957, 7.4974) (-10.8605, 7.4944) (-10.8253, 7.4916) (-10.7902, 7.489) (-10.7552, 7.4865) (-10.7202, 7.4843) (-10.6852, 7.4823) (-10.6503, 7.4805) (-10.6154, 7.4789) (-10.5806, 7.4775) (-10.5459, 7.4763) (-10.5112, 7.4753) (-10.4766, 7.4745) (-10.442, 7.4739) (-10.4075, 7.4735) (-10.3731, 7.4734) (-10.3387, 7.4734) (-10.3044, 7.4737) (-10.2702, 7.4742) (-10.236, 7.4749) (-10.2019, 7.4758) (-10.1679, 7.4769) (-10.134, 7.4783) (-10.1001, 7.4798) (-10.0663, 7.4816) (-10.0326, 7.4836) (-9.9989, 7.4859) (-9.9654, 7.4883) (-9.9319, 7.491) (-9.8985, 7.494) (-9.8652, 7.4971) (-9.832, 7.5006) (-9.7989, 7.5042) (-9.7659, 7.5081) (-9.733, 7.5122) (-9.7002, 7.5166) (-9.6674, 7.5212) (-9.6348, 7.5261) (-9.6023, 7.5312) (-9.5699, 7.5366) (-9.5376, 7.5423) (-9.5055, 7.5483) (-9.4735, 7.5545) (-9.4416, 7.5611) (-9.4098, 7.5679) (-9.3782, 7.5749) (-9.3466, 7.5823) (-9.3152, 7.5899) (-9.284, 7.5977) (-9.2529, 7.606) (-9.222, 7.6147) (-9.1914, 7.6238) (-9.1609, 7.6334) (-9.1307, 7.6434) (-9.1006, 7.6537) (-9.0706, 7.6642) (-9.0408, 7.6748) (-9.0111, 7.6858) (-8.9818, 7.6974) (-8.9529, 7.7099) (-8.9303, 7.7208) (-8.9137, 7.7298) (-8.9029, 7.7361) (-8.8975, 7.7393) knots -1 -1 -1 -1 -1 -1 -0.98571429 -0.97142857 -0.95714286 -0.94285714 -0.92857143 -0.91428571 -0.9 -0.88571429 -0.87142857 -0.85714286 -0.84285714 -0.82857143 -0.81428571 -0.8 -0.78571429 -0.77142857 -0.75714286 -0.74285714 -0.72857143 -0.71428571 -0.7 -0.68571429 -0.67142857 -0.65714286 -0.64285714 -0.62857143 -0.61428571 -0.6 -0.58571429 -0.57142857 -0.55714286 -0.54285714 -0.52857143 -0.51428571 -0.5 -0.48571429 -0.47142857 -0.45714286 -0.44285714 -0.42857143 -0.41428571 -0.4 -0.38571429 -0.37142857 -0.35714286 -0.34285714 -0.32857143 -0.31428571 -0.3 -0.28571429 -0.27142857 -0.25714286 -0.24285714 -0.22857143 -0.21428571 -0.2 -0.18571429 -0.17142857 -0.15714286 -0.14285714 -0.12857143 -0.11428571 -0.1 -0.08571429 -0.07142857 -0.05714286 -0.04285714 -0.02857143 -0.01428571 0 0 0 0 0 0
  line L3 (-8.8975, 7.7393) -> (-8.6674, 7.8767)
  arc A7 (-7.6049, 7.6532) -> (-8.6674, 7.8767) centre (-8.2572, 7.1899) ccw
  arc A8 (-7.6049, 7.6532) -> (-7.4871, 7.491) centre (0, 13.0546) ccw
  arc A9 (-7.6029, 6.4114) -> (-7.4871, 7.491) centre (-8.1292, 7.0139) ccw
  line L4 (-7.6029, 6.4114) -> (-7.8046, 6.2351)
  spline S4 degree 5 poles (-7.8046, 6.2351) (-7.8094, 6.231) (-7.8187, 6.2226) (-7.8323, 6.2096) (-7.8498, 6.1915) (-7.8705, 6.1679) (-7.8906, 6.1436) (-7.9102, 6.1187) (-7.9296, 6.0937) (-7.9488, 6.0684) (-7.9679, 6.043) (-7.9867, 6.0173) (-8.0053, 5.9913) (-8.0234, 5.965) (-8.0412, 5.9383) (-8.0587, 5.9113) (-8.0759, 5.884) (-8.0928, 5.8565) (-8.1095, 5.8287) (-8.126, 5.8008) (-8.1423, 5.7727) (-8.1584, 5.7444) (-8.1742, 5.7159) (-8.1898, 5.6872) (-8.2052, 5.6582) (-8.2203, 5.6291) (-8.2352, 5.5997) (-8.2499, 5.5702) (-8.2645, 5.5405) (-8.2788, 5.5107) (-8.2929, 5.4807) (-8.3068, 5.4505) (-8.3205, 5.4201) (-8.334, 5.3896) (-8.3473, 5.3589) (-8.3604, 5.3281) (-8.3733, 5.2971) (-8.386, 5.2659) (-8.3985, 5.2346) (-8.4109, 5.2032) (-8.423, 5.1716) (-8.435, 5.1398) (-8.4468, 5.108) (-8.4584, 5.076) (-8.4698, 5.0438) (-8.481, 5.0115) (-8.492, 4.9791) (-8.5029, 4.9466) (-8.5135, 4.9139) (-8.524, 4.8811) (-8.5343, 4.8482) (-8.5445, 4.8151) (-8.5544, 4.782) (-8.5642, 4.7487) (-8.5738, 4.7153) (-8.5832, 4.6817) (-8.5924, 4.6481) (-8.6015, 4.6143) (-8.6104, 4.5805) (-8.6191, 4.5465) (-8.6276, 4.5124) (-8.636, 4.4782) (-8.6442, 4.4439) (-8.6522, 4.4094) (-8.66, 4.3749) (-8.6677, 4.3403) (-8.6752, 4.3056) (-8.6825, 4.2707) (-8.6896, 4.2358) (-8.6966, 4.2008) (-8.7034, 4.1657) (-8.7087, 4.1375) (-8.7126, 4.1163) (-8.7152, 4.1022) (-8.7165, 4.0951) knots 0 0 0 0 0 0 0.01428571 0.02857143 0.04285714 0.05714286 0.07142857 0.08571429 0.1 0.11428571 0.12857143 0.14285714 0.15714286 0.17142857 0.18571429 0.2 0.21428571 0.22857143 0.24285714 0.25714286 0.27142857 0.28571429 0.3 0.31428571 0.32857143 0.34285714 0.35714286 0.37142857 0.38571429 0.4 0.41428571 0.42857143 0.44285714 0.45714286 0.47142857 0.48571429 0.5 0.51428571 0.52857143 0.54285714 0.55714286 0.57142857 0.58571429 0.6 0.61428571 0.62857143 0.64285714 0.65714286 0.67142857 0.68571429 0.7 0.71428571 0.72857143 0.74285714 0.75714286 0.77142857 0.78571429 0.8 0.81428571 0.82857143 0.84285714 0.85714286 0.87142857 0.88571429 0.9 0.91428571 0.92857143 0.94285714 0.95714286 0.97142857 0.98571429 1 1 1 1 1 1
  arc A10 (-8.7165, 4.0951) -> (-7.9993, 3.4494) centre (0, 13.0546) ccw
  spline S5 degree 5 poles (-7.9993, 3.4494) (-7.9924, 3.4514) (-7.9786, 3.4554) (-7.958, 3.4615) (-7.9305, 3.4697) (-7.8963, 3.4802) (-7.8622, 3.4908) (-7.8282, 3.5015) (-7.7943, 3.5124) (-7.7606, 3.5235) (-7.7269, 3.5348) (-7.6934, 3.5462) (-7.66, 3.5577) (-7.6267, 3.5695) (-7.5936, 3.5813) (-7.5606, 3.5934) (-7.5277, 3.6056) (-7.495, 3.618) (-7.4623, 3.6305) (-7.4298, 3.6432) (-7.3975, 3.6561) (-7.3652, 3.6691) (-7.3332, 3.6823) (-7.3012, 3.6957) (-7.2694, 3.7092) (-7.2377, 3.7229) (-7.2062, 3.7368) (-7.1748, 3.7508) (-7.1436, 3.765) (-7.1125, 3.7794) (-7.0816, 3.7939) (-7.0508, 3.8086) (-7.0202, 3.8235) (-6.9897, 3.8385) (-6.9594, 3.8537) (-6.9293, 3.8691) (-6.8993, 3.8847) (-6.8695, 3.9004) (-6.8398, 3.9163) (-6.8103, 3.9324) (-6.781, 3.9486) (-6.7519, 3.9651) (-6.723, 3.9817) (-6.6942, 3.9985) (-6.6656, 4.0155) (-6.6372, 4.0326) (-6.609, 4.05) (-6.581, 4.0675) (-6.5532, 4.0852) (-6.5256, 4.1031) (-6.4982, 4.1212) (-6.471, 4.1396) (-6.4441, 4.1581) (-6.4174, 4.1768) (-6.3909, 4.1958) (-6.3646, 4.2149) (-6.3386, 4.2342) (-6.3128, 4.2538) (-6.2872, 4.2735) (-6.2618, 4.2934) (-6.2368, 4.3136) (-6.2121, 4.3341) (-6.1878, 4.3549) (-6.1639, 4.376) (-6.1404, 4.3974) (-6.1171, 4.4191) (-6.0939, 4.4408) (-6.071, 4.4627) (-6.0484, 4.4848) (-6.0263, 4.5073) (-6.005, 4.5305) (-5.9888, 4.5497) (-5.9773, 4.5646) (-5.9699, 4.5747) (-5.9663, 4.5799) knots -1 -1 -1 -1 -1 -1 -0.98571429 -0.97142857 -0.95714286 -0.94285714 -0.92857143 -0.91428571 -0.9 -0.88571429 -0.87142857 -0.85714286 -0.84285714 -0.82857143 -0.81428571 -0.8 -0.78571429 -0.77142857 -0.75714286 -0.74285714 -0.72857143 -0.71428571 -0.7 -0.68571429 -0.67142857 -0.65714286 -0.64285714 -0.62857143 -0.61428571 -0.6 -0.58571429 -0.57142857 -0.55714286 -0.54285714 -0.52857143 -0.51428571 -0.5 -0.48571429 -0.47142857 -0.45714286 -0.44285714 -0.42857143 -0.41428571 -0.4 -0.38571429 -0.37142857 -0.35714286 -0.34285714 -0.32857143 -0.31428571 -0.3 -0.28571429 -0.27142857 -0.25714286 -0.24285714 -0.22857143 -0.21428571 -0.2 -0.18571429 -0.17142857 -0.15714286 -0.14285714 -0.12857143 -0.11428571 -0.1 -0.08571429 -0.07142857 -0.05714286 -0.04285714 -0.02857143 -0.01428571 0 0 0 0 0 0
  line L5 (-5.9663, 4.5799) -> (-5.8121, 4.799)
  arc A11 (-4.7505, 5.0269) -> (-5.8121, 4.799) centre (-5.1579, 4.3385) ccw
  arc A12 (-4.7505, 5.0269) -> (-4.5769, 4.9267) centre (0, 13.0546) ccw
  arc A13 (-4.2435, 3.8934) -> (-4.5769, 4.9267) centre (-4.9694, 4.2297) ccw
  line L6 (-4.2435, 3.8934) -> (-4.3562, 3.6503)
  spline S6 degree 5 poles (-4.3562, 3.6503) (-4.3588, 3.6446) (-4.3639, 3.6331) (-4.3711, 3.6157) (-4.3796, 3.5921) (-4.389, 3.5621) (-4.3974, 3.5317) (-4.4053, 3.501) (-4.4128, 3.4702) (-4.4201, 3.4393) (-4.4271, 3.4083) (-4.4339, 3.3772) (-4.4403, 3.3459) (-4.4461, 3.3145) (-4.4516, 3.2829) (-4.4565, 3.2511) (-4.4611, 3.2192) (-4.4654, 3.1872) (-4.4694, 3.155) (-4.4731, 3.1228) (-4.4765, 3.0905) (-4.4797, 3.0581) (-4.4826, 3.0256) (-4.4852, 2.993) (-4.4874, 2.9603) (-4.4894, 2.9276) (-4.4911, 2.8947) (-4.4925, 2.8617) (-4.4937, 2.8287) (-4.4946, 2.7956) (-4.4953, 2.7624) (-4.4957, 2.7292) (-4.4959, 2.6959) (-4.4958, 2.6625) (-4.4955, 2.6291) (-4.4949, 2.5956) (-4.4941, 2.562) (-4.4931, 2.5284) (-4.4918, 2.4947) (-4.4903, 2.4609) (-4.4885, 2.4271) (-4.4865, 2.3933) (-4.4843, 2.3594) (-4.4819, 2.3254) (-4.4792, 2.2914) (-4.4763, 2.2574) (-4.4732, 2.2233) (-4.4699, 2.1891) (-4.4664, 2.1549) (-4.4626, 2.1207) (-4.4586, 2.0864) (-4.4544, 2.0521) (-4.45, 2.0178) (-4.4454, 1.9834) (-4.4406, 1.949) (-4.4356, 1.9145) (-4.4303, 1.88) (-4.4249, 1.8455) (-4.4192, 1.8109) (-4.4133, 1.7763) (-4.4073, 1.7417) (-4.401, 1.7071) (-4.3945, 1.6724) (-4.3879, 1.6377) (-4.381, 1.603) (-4.3739, 1.5682) (-4.3666, 1.5335) (-4.3591, 1.4987) (-4.3515, 1.4638) (-4.3436, 1.429) (-4.3355, 1.3941) (-4.3289, 1.3662) (-4.3239, 1.3453) (-4.3205, 1.3314) (-4.3187, 1.3244) knots 0 0 0 0 0 0 0.01428571 0.02857143 0.04285714 0.05714286 0.07142857 0.08571429 0.1 0.11428571 0.12857143 0.14285714 0.15714286 0.17142857 0.18571429 0.2 0.21428571 0.22857143 0.24285714 0.25714286 0.27142857 0.28571429 0.3 0.31428571 0.32857143 0.34285714 0.35714286 0.37142857 0.38571429 0.4 0.41428571 0.42857143 0.44285714 0.45714286 0.47142857 0.48571429 0.5 0.51428571 0.52857143 0.54285714 0.55714286 0.57142857 0.58571429 0.6 0.61428571 0.62857143 0.64285714 0.65714286 0.67142857 0.68571429 0.7 0.71428571 0.72857143 0.74285714 0.75714286 0.77142857 0.78571429 0.8 0.81428571 0.82857143 0.84285714 0.85714286 0.87142857 0.88571429 0.9 0.91428571 0.92857143 0.94285714 0.95714286 0.97142857 0.98571429 1 1 1 1 1 1
  arc A14 (-4.3187, 1.3244) -> (-3.4009, 1.0262) centre (0, 13.0546) ccw